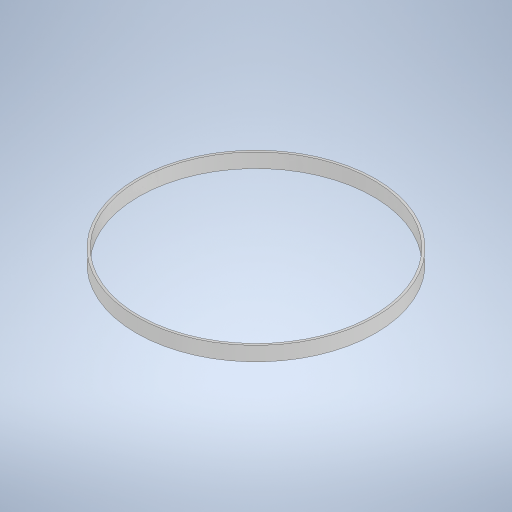
# Autodesk Inventor part: PoleWrap
Saved by Autodesk Inventor 2024.2 (Build 282272000, 272)
## iProperties
Created: 2024-01-15
Part Number: PoleWrap
Material: Aluminum 6061-AHC
Document SubType Name: Modeling
Designer: airso
Density: 2.7 g/cm^3
Appearance: Aluminum - Dark
Author: airso
Autodesk Inventor part; units mm, degrees
ref_plane "YZ Plane" through (0, 0, 0) normal (1, 0, 0) x (0, 1, 0)
ref_plane "XZ Plane" through (0, 0, 0) normal (0, 1, 0) x (-1, 0, 0)
ref_plane "XY Plane" through (0, 0, 0) normal (0, 0, 1) x (1, 0, 0)
sketch "Sketch1" plane through (0, 0, 0) normal (0, 1, 0) x (-1, 0, 0)
  circle A0 centre (0, 0) radius 26.035
  circle A1 centre (0, 0) radius 26.543
  dimension "d0" = 52.07
  dimension "d1" = 0.508
  constraints: 2 centre point, 1 coincident
  measures "d0" diameter of A0
  measures "d1" radial gap between concentric circles of A0 A1
extrude "Extrusion1" add sketch "Sketch1" along normal blind 3.175
body "Solid1"
